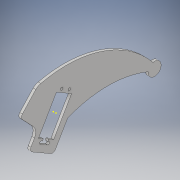
# Autodesk Inventor part: Part3
Saved by Autodesk Inventor 2019 (Build 230136000, 136)
## iProperties
Created: 2023-04-15
Part Number: Part3
Material: Generic
Document SubType Name: Modeling
Designer: Analuam
Density: 1 g/cm^3
Appearance: Default
Author: Analuam
Autodesk Inventor part; units mm, degrees
ref_plane "YZ Plane" through (0, 0, 0) normal (1, 0, 0) x (0, 1, 0)
ref_plane "XZ Plane" through (0, 0, 0) normal (0, 1, 0) x (-1, 0, 0)
ref_plane "XY Plane" through (0, 0, 0) normal (0, 0, 1) x (1, 0, 0)
sketch "Sketch1" plane through (0, 0, 0) normal (1, 0, 0) x (0, 1, 0)
  line L0 (-19.3456, 28.7283) -> (-12.1815, 24.5921)
  line L1 (-11.5536, -13.0731) -> (-35.4981, 0.7513)
  line L2 (-36.9622, 6.2154) -> (-24.8097, 27.2642)
  line L3 (-0.2893, 26.0068) -> (12.8245, 38.4809)
  arc A0 (-19.3456, 28.7283) -> (-24.8097, 27.2642) centre (-21.3456, 25.2642) ccw
  arc A1 (-12.1815, 24.5921) -> (-0.2893, 26.0068) centre (-7.1815, 33.2523) ccw
  line L4 (18.2952, 38.5212) -> (34.9263, 23.1612)
  arc A2 (18.2952, 38.5212) -> (12.8245, 38.4809) centre (15.5813, 35.5827) ccw
  arc A3 (38.0158, 17.396) -> (34.9263, 23.1612) centre (28.1415, 15.815) ccw
  line L5 (-14.9818, 20.1875) -> (20.5253, -0.3125)
  line L6 (20.5253, -0.3125) -> (10.5253, -17.633)
  line L7 (10.5253, -17.633) -> (-24.9818, 2.867)
  circle A4 centre (20.9698, -6.3427) radius 1.5
  circle A5 centre (15.9698, -15.0029) radius 1.5
  arc A6 (-19.1272, 16.8073) -> (-21.727, 18.3044) centre (-20.4271, 17.5559) ccw
  arc A7 (-26.7253, 9.6471) -> (-24.1272, 8.1471) centre (-25.4262, 8.8971) ccw
  line L8 (-21.7318, 8.4961) -> (-23.3772, 9.4461)
  line L9 (-24.9818, 2.867) -> (-21.7318, 8.4961)
  line L10 (-18.2318, 14.5583) -> (-14.9818, 20.1875)
  line L11 (-26.7253, 9.6471) -> (-21.7253, 18.3073)
  line L12 (-19.8772, 15.5083) -> (-18.2318, 14.5583)
  line L13 (-19.1272, 16.8073) -> (-19.8772, 15.5083)
  line L14 (-23.3772, 9.4461) -> (-24.1272, 8.1471)
  arc A8 (-11.5536, -105.0286) -> (-5.2043, -110.6419) centre (-12.4778, -112.4714) ccw
  arc A9 (-11.5536, -105.0286) -> (-11.5536, -13.0731) centre (-124.6127, -59.0508) ccw
  arc A10 (-5.2043, -110.6419) -> (38.0158, 17.396) centre (-86.2024, -11.9868) ccw
  arc A11 (-36.9622, 6.2154) -> (-35.4981, 0.7513) centre (-33.4981, 4.2154) ccw
  circle A12 centre (-11.8158, 5.9264) radius 2.6887
  line L15 (-11.8447, 5.8764) -> (38.9266, -23.4364)
  line L16 (38.9266, -23.4364) -> (-12.4778, -112.4714)
  line L17 (-12.4778, 5.8764) -> (-12.4778, -112.4714)
  point P0 (0, 0)
  point P1 (22.6035, 14.6658)
  point P2 (37.4247, 20.8538)
  dimension "d15" = 4
  dimension "d16" = 10
  dimension "d20" = 4
  dimension "d22" = 10
  dimension "d24" = 41
  dimension "d25" = 20
  dimension "d27" = 3.4
  dimension "d36" = 15
  dimension "d37" = 4
  dimension "d40" = 90
  constraints: 36 end point, 21 point on circle, 13 centre point, 9 tangent, 5 parallel, 2 perpendicular, 2 point on line
  measures "d15" radius of A0
  measures "d16" radius of A1
  measures "d20" radius of A2
  measures "d22" radius of A3
  measures "d24" distance of L6.end L7.end
  measures "d25" distance of L5.end L6.end
  measures "d27" distance from line of L6 A4.centre
  measures "d36" diameter of A8
  measures "d37" radius of A11
  measures "d40" angle of L16 L15
sketch "Sketch2" plane through (0, 0, 0) normal (1, 0, 0) x (0, 1, 0)
  point P0 (0, 0)
extrude "Extrusion1" add sketch "Sketch1" along normal blind 3 contours L0 A1 L3 A2 L4 A3 A10 A8 L17 L16 L15 L6 L5 L10 L12 L13 A6 L11 A7 L14 L8 L9 L7 L1 A11 L2 A0 | L17 L7 L6 L15 L16 A8 A9 L1
sketch "Sketch3" plane through (3, 0, 0) normal (1, 0, 0) x (0, 0, -1)
  point P0 (0, 0)
body "Solid1"
